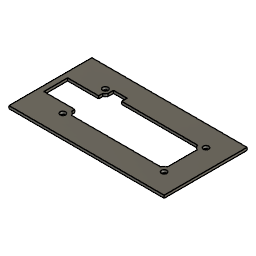
FInalControllerPrototype (Autodesk Fusion 360 archive; units mm, degrees)
design "LCD_Holder"
part number: 2026-04-03-21-14-27-692
Autodesk Fusion 360 part; units mm, degrees
note: some values were not read from the file. Chosen so that the rebuilt part matches the saved one: which pieces of a blend or face edit are solid.
sketch "Sketch1" plane through (0, 0, 0) normal (0, 0, 1) x (1, 0, 0)
  line L0 (0, 0) -> (-37, 0) construction
  line L1 (-37, 0) -> (-37, -15) construction
  line L2 (0, 0) -> (38, 0) construction
  line L3 (38, 0) -> (38, -15) construction
  line L4 (-37, 0) -> (-37, 16.5) construction
  line L5 (38, 0) -> (38, 16) construction
  circle A0 centre (-37, 16.5) radius 2
  circle A1 centre (38, 16) radius 2
  circle A2 centre (38, -15) radius 2
  circle A3 centre (-37, -15) radius 2
  line L6 (-37, 16.5) -> (-37, 31.5) construction
  line L7 (-37, 31.5) -> (-62, 31.5) construction
  line L8 (38, -15) -> (53, -15) construction
  line L9 (53, -15) -> (53, -30) construction
  line L10 (-62, 31.5) -> (53, 31.5)
  line L11 (53, 31.5) -> (53, -30)
  line L12 (53, -30) -> (-62, -30)
  line L13 (-62, -30) -> (-62, 31.5)
  line L14 (-37, 16.5) -> (-35, 16.5) construction
  line L15 (-35, 16.5) -> (-35, 14.5) construction
  line L16 (38, -15) -> (36, -15) construction
  line L17 (36, -15) -> (36, -13) construction
  line L18 (-35, 14.5) -> (36, 14.5)
  line L19 (36, 14.5) -> (36, -13)
  line L20 (36, -13) -> (-35, -13)
  line L21 (-35, -13) -> (-35, 14.5)
  line L22 (-35, 14.5) -> (-35, 9.5) construction
  line L23 (-35, -13) -> (-35, -8) construction
  line L24 (-35, 9.5) -> (-62, 9.5)
  line L25 (-35, -8) -> (-62, -8)
  line L26 (-35, -8) -> (-58, -8) construction
  line L27 (-58, -8) -> (-58, 9.5)
  line L28 (-35, 14.5) -> (-33, 14.5) construction
  line L29 (-33, 14.5) -> (-33, 18.5)
  line L30 (-33, 18.5) -> (-23, 18.5)
  line L31 (-23, 18.5) -> (-23, 14.5)
  circle A4 centre (-37, -15) radius 5
  circle A5 centre (38, -15) radius 5
  circle A6 centre (38, 16) radius 5
  circle A7 centre (-37, 16.5) radius 4.4721
  dimension "d19" = 37
  dimension "d20" = 38
  dimension "d21" = 15
  dimension "d22" = 16.5
  dimension "d23" = 16
  dimension "d24" = 4
  dimension "d25" = 4
  dimension "d26" = 4
  dimension "d27" = 4
  dimension "d28" = 15
  dimension "d29" = 25
  dimension "d30" = 15
  dimension "d31" = 15
  dimension "d32" = 2
  dimension "d33" = 2
  dimension "d34" = 2
  dimension "d35" = 2
  dimension "d36" = 5
  dimension "d37" = 5
  dimension "d40" = 23
  dimension "d41" = 2
  dimension "d42" = 4
  dimension "d43" = 10
  dimension "d44" = 10
  dimension "d45" = 10
  dimension "d46" = 10
  constraint coincident L0.start L2.start
  constraint parallel L0 L2
  constraint perpendicular L2 L3
  constraint perpendicular L0 L4
  constraint perpendicular L2 L5
  constraint coincident L4.end A0.centre
  constraint coincident L5.end A1.centre
  constraint coincident L3.end A2.centre
  constraint coincident L1.end A3.centre
  constraint parallel L4 L6
  constraint perpendicular L6 L7
  constraint perpendicular L3 L8
  constraint perpendicular L8 L9
  constraint horizontal L10
  constraint vertical L11
  constraint horizontal L12
  constraint vertical L13
  constraint perpendicular L6 L14
  constraint perpendicular L14 L15
  constraint perpendicular L3 L16
  constraint perpendicular L16 L17
  constraint horizontal L18
  constraint vertical L19
  constraint horizontal L20
  constraint vertical L21
  constraint perpendicular L18 L22
  constraint perpendicular L20 L23
  constraint coincident L13 L24.end
  constraint perpendicular L13 L24
  constraint coincident L13 L25.end
  constraint perpendicular L13 L25
  constraint perpendicular L1 L26
  constraint coincident L24 L27.end
  constraint perpendicular L24 L27
  constraint perpendicular L22 L28
  constraint perpendicular L18 L29
  constraint perpendicular L29 L30
  constraint coincident L18 L31.end
  constraint perpendicular L18 L31
  constraint concentric A3 A4
  constraint concentric A1 A6
  constraint concentric A0 A7
  constraint coincident L28.end A7
  measures "d19" distance of L0.start L0.end
  measures "d20" distance of L0.start L2.end
  measures "d21" distance of L2.end L3.end
  measures "d22" distance of L0.end L4.end
  measures "d23" distance of L2.end L5.end
  measures "d24" diameter of A0
  measures "d25" diameter of A1
  measures "d26" diameter of A2
  measures "d27" diameter of A3
  measures "d28" distance of L4.end L6.end
  measures "d29" distance of L6.end L7.end
  measures "d30" distance of L3.end L8.end
  measures "d31" distance of L8.end L9.end
  measures "d32" distance of L4.end L14.end
  measures "d33" distance of L14.end L15.end
  measures "d34" distance of L3.end L16.end
  measures "d35" distance of L16.end L17.end
  measures "d36" distance of L15.end L22.end
  measures "d37" distance of L20.end L23.end
  measures "d40" distance of L23.end L26.end
  measures "d41" distance of L15.end L28.end
  measures "d42" distance of L28.end L29.end
  measures "d43" distance of L29.end L30.end
  measures "d44" diameter of A4
  measures "d45" diameter of A5
  measures "d46" diameter of A6
extrude "Extrude3" add sketch "Sketch1" along normal blind 2 contours L10 L11 L12 L13 L18 L19 L20 L21 L24 L25 L30 L31 A4 A5 A6 A7 | L13 L24 L25 L27 | L18 L21 L29 A7 | L18 L21 A7 | L20 L21 A4 | L20 L21 A4 | L19 L20 A5 | L19 L20 A5 | L18 L19 A6 | L18 L19 A6
equation "d40 = 27 mm - 4 mm"
named bodies: "LCD_Holder"

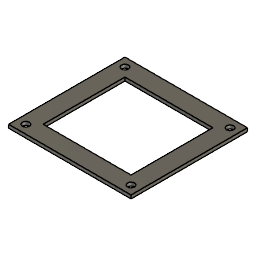
design "ESP_Screws"
part number: 2026-04-04-21-19-26-953
Autodesk Fusion 360 part; units mm, degrees
sketch "Sketch1" plane through (0, 0, 0) normal (0, 0, 1) x (1, 0, 0)
  line L0 (30.25, 28.5) -> (-30.25, 28.5) construction
  line L1 (-30.25, 28.5) -> (-30.25, -28.5) construction
  line L2 (-30.25, -28.5) -> (30.25, -28.5) construction
  line L3 (30.25, -28.5) -> (30.25, 28.5) construction
  line L4 (30.25, 28.5) -> (-30.25, -28.5) construction
  line L5 (-30.25, 28.5) -> (30.25, -28.5) construction
  circle A0 centre (-30.25, 28.5) radius 2
  circle A1 centre (30.25, 28.5) radius 2
  circle A2 centre (-30.25, -28.5) radius 2
  circle A3 centre (30.25, -28.5) radius 2
  line L6 (-30.25, 28.5) -> (-30.25, 33.5) construction
  line L7 (-30.25, 33.5) -> (-35.25, 33.5) construction
  line L8 (30.25, -28.5) -> (35.25, -28.5) construction
  line L9 (35.25, -28.5) -> (35.25, -33.5) construction
  line L10 (-35.25, 33.5) -> (35.25, 33.5)
  line L11 (35.25, 33.5) -> (35.25, -33.5)
  line L12 (35.25, -33.5) -> (-35.25, -33.5)
  line L13 (-35.25, -33.5) -> (-35.25, 33.5)
  line L14 (-30.25, 28.5) -> (-25.25, 28.5) construction
  line L15 (-25.25, 28.5) -> (-25.25, 23.5) construction
  line L16 (30.25, -28.5) -> (30.25, -23.5) construction
  line L17 (30.25, -23.5) -> (25.25, -23.5) construction
  line L18 (-25.25, 23.5) -> (25.25, 23.5)
  line L19 (25.25, 23.5) -> (25.25, -23.5)
  line L20 (25.25, -23.5) -> (-25.25, -23.5)
  line L21 (-25.25, -23.5) -> (-25.25, 23.5)
  dimension "d1" = 60.5
  dimension "d2" = 57
  dimension "d3" = 4
  dimension "d4" = 4
  dimension "d5" = 4
  dimension "d6" = 4
  dimension "d7" = 5
  dimension "d10" = 5
  constraint horizontal L0
  constraint perpendicular L0 L1
  constraint parallel L0 L2
  constraint parallel L1 L3
  constraint coincident L4 origin
  constraint coincident L5 origin
  constraint coincident L0.end L1.start
  constraint coincident L0.start L3.end
  constraint coincident L1.end L2.start
  constraint coincident L2.end L3.start
  constraint perpendicular L0 L6
  constraint perpendicular L6 L7
  constraint equal L6 L7
  constraint perpendicular L3 L8
  constraint perpendicular L8 L9
  constraint equal L6 L8
  constraint equal L8 L9
  constraint horizontal L10
  constraint vertical L11
  constraint horizontal L12
  constraint vertical L13
  constraint coincident L0 L14.end
  constraint perpendicular L14 L15
  constraint coincident L3 L16.end
  constraint perpendicular L16 L17
  constraint equal L14 L15
  constraint equal L15 L17
  constraint equal L16 L17
  constraint horizontal L18
  constraint vertical L19
  constraint horizontal L20
  constraint vertical L21
  measures "d1" distance of L1.end L2.end
  measures "d2" distance of L0.end L1.end
  measures "d3" diameter of A0
  measures "d4" diameter of A1
  measures "d5" diameter of A2
  measures "d6" diameter of A3
  measures "d7" distance of L0.end L6.end
  measures "d10" distance of L0.end L14.end
extrude "Extrude1" add sketch "Sketch1" along normal blind 2
named bodies: "ESP_Screws"

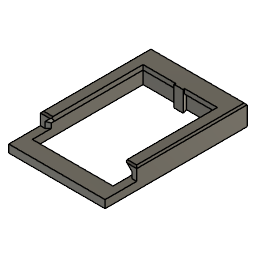
design "Keypad_Top"
part number: 2026-04-03-21-53-20-914
Autodesk Fusion 360 part; units mm, degrees
sketch "Sketch1" plane through (0, 0, 0) normal (0, 0, 1) x (1, 0, 0)
  line L0 (25.5, 5) -> (-25.5, 5)
  line L1 (-25.5, 5) -> (-25.5, -5)
  line L2 (-25.5, -5) -> (25.5, -5)
  line L3 (25.5, -5) -> (25.5, 5)
  line L4 (25.5, 5) -> (-25.5, -5) construction
  line L5 (-25.5, 5) -> (25.5, -5) construction
  line L6 (-25.5, -5) -> (-3, -5) construction
  line L7 (25.5, -5) -> (3, -5) construction
  line L8 (-25.5, 5) -> (-30.5, 5)
  line L9 (-30.5, 5) -> (-30.5, -65)
  line L10 (-30.5, -65) -> (-25.5, -65)
  line L11 (-25.5, -65) -> (-25.5, 5)
  line L12 (25.5, 5) -> (30.5, 5)
  line L13 (30.5, 5) -> (30.5, -65)
  line L14 (30.5, -65) -> (25.5, -65)
  line L15 (25.5, -65) -> (25.5, 5)
  line L16 (-3, -5) -> (-3, -8) construction
  line L17 (3, -5) -> (3, -8) construction
  line L18 (-3, -5) -> (-2, -5) construction
  line L19 (3, -5) -> (2, -5) construction
  line L20 (-2, -5) -> (-3, -8)
  line L21 (-3, -8) -> (3, -8)
  line L22 (3, -8) -> (2, -5)
  dimension "d1" = 51
  dimension "d2" = 10
  dimension "d3" = 22.5
  dimension "d5" = 5
  dimension "d6" = 70
  dimension "d9" = 3
  dimension "d11" = 1
  constraint horizontal L0
  constraint perpendicular L0 L1
  constraint parallel L0 L2
  constraint parallel L1 L3
  constraint coincident L4 origin
  constraint coincident L5 origin
  constraint perpendicular L1 L6
  constraint perpendicular L3 L7
  constraint horizontal L8
  constraint vertical L9
  constraint horizontal L10
  constraint vertical L11
  constraint horizontal L12
  constraint vertical L13
  constraint horizontal L14
  constraint vertical L15
  constraint perpendicular L6 L16
  constraint perpendicular L2 L17
  constraint coincident L2 L18.end
  constraint perpendicular L17 L19
  constraint equal L11 L15
  constraint equal L6 L7
  constraint equal L16 L17
  constraint equal L8 L12
  measures "d1" distance of L1.end L2.end
  measures "d2" distance of L0.end L1.end
  measures "d3" distance of L1.end L6.end
  measures "d5" distance of L0.end L8.end
  measures "d6" distance of L0.end L10.end
  measures "d9" distance of L6.end L16.end
  measures "d11" distance of L7.end L19.end
extrude "Extrude1" add sketch "Sketch1" along normal blind 8
sketch "Sketch2" plane through (0, 0, 0) normal (0, 0, 1) x (1, 0, 0)
  line L0 (30.5, 5) -> (-31, 5)
  line L1 (-30.5, 5) -> (30.5, 5)
  line L2 (30.5, 5) -> (30.5, -85)
  line L3 (30.5, -85) -> (-30.5, -85)
  line L4 (-30.5, -85) -> (-30.5, 5)
  line L5 (-30.5, -85) -> (30.5, -85)
  line L6 (-25.5, -5) -> (25.5, -5)
  line L7 (25.5, -5) -> (25.5, -75)
  line L8 (25.5, -75) -> (-25.5, -75)
  line L9 (-25.5, -75) -> (-25.5, -5)
  line L10 (30.5, 5) -> (-30.5, 5)
  line L11 (-30.5, 5) -> (-30.5, -65)
  line L12 (-30.5, -65) -> (-25.5, -65)
  line L13 (-25.5, -65) -> (-25.5, -5)
  line L14 (-25.5, -5) -> (-2, -5)
  line L15 (-2, -5) -> (-3, -8)
  line L16 (-3, -8) -> (3, -8)
  line L17 (3, -8) -> (2, -5)
  line L18 (2, -5) -> (25.5, -5)
  line L19 (25.5, -5) -> (25.5, -65)
  line L20 (25.5, -65) -> (30.5, -65)
  line L21 (30.5, -65) -> (30.5, 5)
  point P0 (-30.5, 5)
  point P1 (30.5, 5)
  point P2 (-25.5, -5)
  point P3 (25.5, -5)
  dimension "d31" = 90
  dimension "d45" = 70
  constraint horizontal L0
  constraint horizontal L1
  constraint vertical L2
  constraint horizontal L3
  constraint vertical L4
  constraint horizontal L5
  constraint coincident L0.end L1
  constraint coincident P0 L1.start
  constraint coincident L0.start L1.end
  constraint coincident L2.end L3.start
  constraint horizontal L6
  constraint vertical L7
  constraint horizontal L8
  constraint vertical L9
  constraint coincident P2 L6.start
  measures "d31" distance of P0 L3.end
  measures "d45" distance of P2 L8.end
extrude "Extrude2" add sketch "Sketch2" against normal blind 5 contours L0 L1 L2 L4 L6 L7 L9 L10 L11 L12 L13 L14 L18 L19 L20 L21 | L2 L3 L4 L5 L7 L8 L9 L12 L20 | L6 L15 L16 L17
ref_plane "WorkPlane1" through (0, -75, 3) normal (0, 0, 1) x (1, 0, 0)
sketch "Sketch4" plane through (0, 0, 3) normal (0, 0, 1) x (1, 0, 0)
  line L0 (-25.5, -65) -> (-23.5, -65) construction
  line L1 (25.5, -65) -> (23.5, -65) construction
  line L2 (-25.5, -5) -> (-25.5, -7) construction
  line L3 (-23.5, -65) -> (-25.5, -65)
  line L4 (-25.5, -65) -> (-25.5, -5)
  line L5 (-25.5, -5) -> (-23.5, -5)
  line L6 (-23.5, -5) -> (-23.5, -65)
  line L7 (23.5, -65) -> (25.5, -65)
  line L8 (25.5, -65) -> (25.5, -5)
  line L9 (25.5, -5) -> (23.5, -5)
  line L10 (23.5, -5) -> (23.5, -65)
  line L11 (-25.5, -7) -> (25.5, -7)
  line L12 (25.5, -7) -> (25.5, -5)
  line L13 (25.5, -5) -> (-25.5, -5)
  line L14 (-25.5, -5) -> (-25.5, -7)
  point P0 (-25.5, -65)
  point P1 (-25.5, -5)
  point P2 (25.5, -5)
  dimension "d17" = 2
  dimension "d18" = 2
  dimension "d19" = 2
  constraint horizontal L0
  constraint horizontal L1
  constraint vertical L2
  constraint horizontal L3
  constraint vertical L4
  constraint horizontal L5
  constraint vertical L6
  constraint horizontal L7
  constraint vertical L8
  constraint horizontal L9
  constraint vertical L10
  constraint horizontal L11
  constraint vertical L12
  constraint horizontal L13
  constraint vertical L14
  constraint coincident P0 L0.start
  constraint coincident P1 L2.start
  constraint coincident P2 L8.end
  constraint equal L6 L10
  measures "d17" distance of P0 L0.end
  measures "d18" distance of L1.start L1.end
  measures "d19" distance of P1 L2.end
extrude "Extrude3" add sketch "Sketch4" along normal blind 5
chamfer "Chamfer1" distance 2 angle 45 4 edges at (-23.5, -36, 3) (-13.0833, -7, 3) (13.0833, -7, 3) (23.5, -36, 3)
chamfer "Chamfer2" distance 1 angle 45 5 edges at (30.5, -30, 8) (0, 5, 8) (-30.5, -30, 8) (27, -65, 8) (-27, -65, 8)
chamfer "Chamfer3" distance 2 angle 45 4 edges at (-25.5, -65, 1.5) (-24.5, -65, 4) (25.5, -65, 1.5) (24.5, -65, 4)
named bodies: "Keypad_Top"

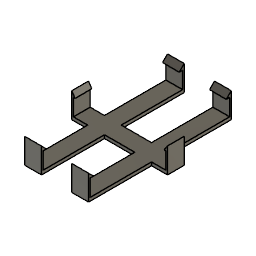
design "Breadboard_Holder"
part number: 2026-04-04-21-55-53-207
Autodesk Fusion 360 part; units mm, degrees
sketch "Sketch1" plane through (0, 0, 0) normal (0, 0, 1) x (1, 0, 0)
  line L0 (27.5, 5) -> (-27.5, 5)
  line L1 (-27.5, 5) -> (-27.5, -5)
  line L2 (-27.5, -5) -> (27.5, -5)
  line L3 (27.5, -5) -> (27.5, 5)
  line L4 (27.5, 5) -> (-27.5, -5) construction
  line L5 (-27.5, 5) -> (27.5, -5) construction
  line L6 (-27.5, 5) -> (-28.5, 5)
  line L7 (-28.5, 5) -> (-28.5, -5)
  line L8 (-28.5, -5) -> (-27.5, -5)
  line L9 (-27.5, -5) -> (-27.5, 5)
  line L10 (27.5, 5) -> (28.5, 5)
  line L11 (28.5, 5) -> (28.5, -5)
  line L12 (28.5, -5) -> (27.5, -5)
  line L13 (27.5, -5) -> (27.5, 5)
  dimension "d1" = 55
  dimension "d2" = 10
  dimension "d3" = 1
  dimension "d4" = 1
  constraint horizontal L0
  constraint perpendicular L0 L1
  constraint parallel L0 L2
  constraint parallel L1 L3
  constraint coincident L4 origin
  constraint coincident L5 origin
  constraint horizontal L6
  constraint vertical L7
  constraint horizontal L8
  constraint vertical L9
  constraint horizontal L10
  constraint vertical L11
  constraint horizontal L12
  constraint vertical L13
  measures "d1" distance of L1.end L2.end
  measures "d2" distance of L0.end L1.end
  measures "d3" distance of L0.end L6.end
  measures "d4" distance of L0.start L10.end
extrude "Extrude1" add sketch "Sketch1" along normal blind 2
sketch "Sketch2" plane through (0, 0, 2) normal (0, 0, 1) x (-1, 0, 0)
  line L0 (-28.5, -5) -> (28.5, -5)
  line L1 (28.5, -5) -> (28.5, 5)
  line L2 (28.5, 5) -> (-28.5, 5)
  line L3 (-28.5, 5) -> (-28.5, -5)
  line L4 (-27.5, -5) -> (27.5, -5)
  line L5 (27.5, -5) -> (27.5, 5)
  line L6 (27.5, 5) -> (-27.5, 5)
  line L7 (-27.5, 5) -> (-27.5, -5)
  line L8 (-27.5, -5) -> (27.5, 5) construction
  line L9 (27.5, -5) -> (-27.5, 5) construction
  dimension "d7" = 55
  constraint horizontal L4
  constraint perpendicular L4 L5
  constraint parallel L4 L6
  constraint parallel L5 L7
  constraint coincident L8 origin
  constraint coincident L9 origin
  measures "d7" distance of L5.end L6.end
extrude "Extrude2" add sketch "Sketch2" along normal blind 10 contours L0 L2 L3 L7 | L0 L1 L2 L5
sketch "Sketch3" plane through (0, 0, 12) normal (0, 0, 1) x (-1, 0, 0)
  line L0 (28.5, -5) -> (28.5, 5)
  line L1 (28.5, 5) -> (27.5, 5)
  line L2 (27.5, 5) -> (27.5, -5)
  line L3 (27.5, -5) -> (28.5, -5)
  line L4 (28.5, -5) -> (26.5, -5)
  line L5 (26.5, -5) -> (26.5, 5)
  line L6 (26.5, 5) -> (28.5, 5)
  line L7 (28.5, 5) -> (28.5, -5)
  dimension "d10" = 2
  constraint horizontal L4
  constraint vertical L5
  constraint horizontal L6
  constraint vertical L7
  constraint coincident L0.start L3.end
  measures "d10" distance of L0.start L4.end
extrude "Extrude3" add sketch "Sketch3" along normal blind 3
sketch "Sketch5" plane through (0, -5, 0) normal (0, -1, 0) x (1, 0, 0)
  line L0 (-28.5, 0) -> (28.5, 0)
  line L1 (28.5, 0) -> (28.5, 12)
  line L2 (28.5, 12) -> (27.5, 12)
  line L3 (27.5, 12) -> (27.5, 2)
  line L4 (27.5, 2) -> (-27.5, 2)
  line L5 (-27.5, 2) -> (-27.5, 12)
  line L6 (-27.5, 12) -> (-26.5, 12)
  line L7 (-26.5, 12) -> (-26.5, 15)
  line L8 (-26.5, 15) -> (-28.5, 15)
  line L9 (-28.5, 15) -> (-28.5, 0)
  line L10 (-26.5, 12) -> (-28.5, 15)
  constraint coincident L6.end L7.start
  constraint coincident L8.end L9.start
extrude "Extrude4" cut sketch "Sketch5" against normal blind 10 contours L7 L8 L10
mirror "Mirror2" about plane through (0, 0, 0) normal (1, 0, 0) of "Extrude3", "Extrude4"
sketch "Sketch6" plane through (0, 0, 0) normal (0, 0, 1) x (1, 0, 0)
  line L0 (-9, 41.5) -> (-19, 41.5)
  line L1 (-19, 41.5) -> (-19, -41.5)
  line L2 (-19, -41.5) -> (-9, -41.5)
  line L3 (-9, -41.5) -> (-9, 41.5)
  line L4 (-9, 41.5) -> (-19, -41.5) construction
  line L5 (-19, 41.5) -> (-9, -41.5) construction
  line L6 (-19, 41.5) -> (-9, 41.5)
  line L7 (-9, 41.5) -> (-9, 42.5)
  line L8 (-9, 42.5) -> (-19, 42.5)
  line L9 (-19, 42.5) -> (-19, 41.5)
  line L10 (-19, -41.5) -> (-9, -41.5)
  line L11 (-9, -41.5) -> (-9, -42.5)
  line L12 (-9, -42.5) -> (-19, -42.5)
  line L13 (-19, -42.5) -> (-19, -41.5)
  dimension "d19" = 10
  dimension "d20" = 83
  dimension "d21" = 1
  dimension "d22" = 1
  constraint horizontal L0
  constraint perpendicular L0 L1
  constraint parallel L0 L2
  constraint parallel L1 L3
  constraint horizontal L6
  constraint vertical L7
  constraint horizontal L8
  constraint vertical L9
  constraint horizontal L10
  constraint vertical L11
  constraint horizontal L12
  constraint vertical L13
  measures "d19" distance of L1.end L2.end
  measures "d20" distance of L0.end L1.end
  measures "d21" distance of L0.end L8.end
  measures "d22" distance of L1.end L12.end
extrude "Extrude5" add sketch "Sketch6" along normal blind 2
mirror "Mirror4" about plane through (0, 0, 0) normal (1, 0, 0) of "Extrude5"
sketch "Sketch10" plane through (0, 0, 2) normal (0, 0, 1) x (-1, 0, 0)
  line L0 (-19, 5) -> (-27.5, 5)
  line L1 (-27.5, 5) -> (-27.5, -5)
  line L2 (-27.5, -5) -> (-19, -5)
  line L3 (-19, -5) -> (-19, -42.5)
  line L4 (-19, -42.5) -> (-9, -42.5)
  line L5 (-9, -42.5) -> (-9, -5)
  line L6 (-9, -5) -> (9, -5)
  line L7 (9, -5) -> (9, -42.5)
  line L8 (9, -42.5) -> (19, -42.5)
  line L9 (19, -42.5) -> (19, -5)
  line L10 (19, -5) -> (27.5, -5)
  line L11 (27.5, -5) -> (27.5, 5)
  line L12 (27.5, 5) -> (19, 5)
  line L13 (19, 5) -> (19, 42.5)
  line L14 (19, 42.5) -> (9, 42.5)
  line L15 (9, 42.5) -> (9, 5)
  line L16 (9, 5) -> (-9, 5)
  line L17 (-9, 5) -> (-9, 42.5)
  line L18 (-9, 42.5) -> (-19, 42.5)
  line L19 (-19, 42.5) -> (-19, 5)
  line L20 (19, -42.5) -> (9, -42.5)
  line L21 (9, -42.5) -> (9, -41.5)
  line L22 (9, -41.5) -> (19, -41.5)
  line L23 (19, -41.5) -> (19, -42.5)
  dimension "d37" = 1
  constraint horizontal L20
  constraint vertical L21
  constraint horizontal L22
  constraint vertical L23
  constraint coincident L8.end L9.start
  measures "d37" distance of L8.end L22.end
extrude "Extrude9" add sketch "Sketch10" along normal blind 10 contours L7 L8 L9 L20 L21 L22 L23
sketch "Sketch11" plane through (0, 0, 12) normal (0, 0, 1) x (-1, 0, 0)
  line L0 (19, -41.5) -> (9, -41.5)
  line L1 (9, -41.5) -> (9, -42.5)
  line L2 (9, -42.5) -> (19, -42.5)
  line L3 (19, -42.5) -> (19, -41.5)
  line L4 (19, -42.5) -> (9, -42.5)
  line L5 (9, -42.5) -> (9, -39.5)
  line L6 (9, -39.5) -> (19, -39.5)
  line L7 (19, -39.5) -> (19, -42.5)
  dimension "d40" = 3
  constraint horizontal L4
  constraint vertical L5
  constraint horizontal L6
  constraint vertical L7
  constraint coincident L2.end L3.start
  measures "d40" distance of L2.end L6.end
extrude "Extrude10" add sketch "Sketch11" along normal blind 3
sketch "Sketch12" plane through (-19, 0, 0) normal (-1, 0, 0) x (0, -1, 0)
  line L0 (-5, 0) -> (-5, 2)
  line L1 (-5, 2) -> (-41.5, 2)
  line L2 (-41.5, 2) -> (-41.5, 12)
  line L3 (-41.5, 12) -> (-39.5, 12)
  line L4 (-39.5, 12) -> (-39.5, 15)
  line L5 (-39.5, 15) -> (-42.5, 15)
  line L6 (-42.5, 15) -> (-42.5, 0)
  line L7 (-42.5, 0) -> (-5, 0)
  line L8 (-39.5, 12) -> (-42.5, 15)
  constraint coincident L3.end L4.start
  constraint coincident L5.end L6.start
extrude "Extrude11" cut sketch "Sketch12" against normal blind 10 contours L4 L5 L8
mirror "Mirror5" about plane through (0, 0, 0) normal (1, 0, 0) of "Extrude9", "Extrude10", "Extrude11"
mirror "Mirror6" about plane through (0, 0, 0) normal (0, 1, 0) of "Extrude9", "Extrude10", "Extrude11", "Mirror5"
named bodies: "Breadboard_Holder"
